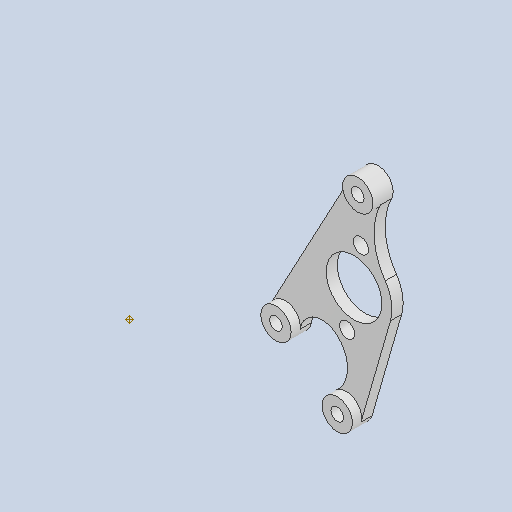
# Autodesk Inventor part: モータマウント
Saved by Autodesk Inventor 2023 (Build 270158030, 158C)
## iProperties
Created: 2022-01-29
Part Number: モータマウント
Material: Aluminum 2014-T4
Document SubType Name: Modeling
Designer: acps
Density: 2.8 g/cm^3
Appearance: Satin
Author: acps
Autodesk Inventor part; units mm, degrees
ref_plane "YZ Plane" through (0, 0, 0) normal (1, 0, 0) x (0, 1, 0)
ref_plane "XZ Plane" through (0, 0, 0) normal (0, 1, 0) x (-1, 0, 0)
ref_plane "XY Plane" through (0, 0, 0) normal (0, 0, 1) x (1, 0, 0)
sketch "Sketch1" plane through (0, 0, 0) normal (0, 0, 1) x (1, 0, 0)
  circle A0 centre (46.616, 30) radius 5.5
  circle A1 centre (49.1519, 48.073) radius 1.25
  circle A2 centre (45.1, 8.5) radius 1.25
  circle A3 centre (47.9747, 37.8838) radius 1.5
  line L0 (47.9747, 37.8838) -> (46.616, 30)
  line L1 (46.616, 30) -> (45.2573, 22.1162)
  circle A4 centre (45.2573, 22.1162) radius 2.75 construction
  circle A5 centre (33, 18) radius 1.25
  arc A6 (53.8224, 27.9221) -> (52.7865, 34.2633) centre (46.616, 30) ccw
  circle A7 centre (45.2573, 22.1162) radius 1.5
  circle A8 centre (49.1519, 48.073) radius 3
  circle A9 centre (33, 18) radius 3
  circle A10 centre (45.1, 8.5) radius 3
  arc A11 (51.8473, 46.7559) -> (52.7865, 34.2633) centre (62.9884, 41.3118) ccw
  arc A12 (43.1426, 10.7734) -> (43.3656, 20.1202) centre (39.0319, 15.5476) ccw
  arc A13 (43.3656, 20.1202) -> (35.9679, 17.5623) centre (40.3315, 16.9188) ccw
  line L2 (53.8224, 27.9221) -> (47.9826, 7.6688)
  line L3 (46.509, 49.4925) -> (30.3571, 19.4195)
  circle A14 centre (47.9747, 37.8838) radius 3 construction
  point P0 (0, 0)
  point P1 (0, 0)
  dimension "d65" = 5.5
  dimension "d61" = 11
  dimension "d62" = 3
  dimension "d63" = 8
  dimension "d64" = 8
  dimension "d66" = 2
  dimension "d67" = 3
  dimension "d68" = 6
  dimension "d69" = 6
  dimension "d70" = 6
  dimension "d71" = 6.3
  dimension "d72" = 12.4
  dimension "d73" = 1.5
  constraints: 14 centre point, 14 point on circle, 9 tangent, 8 end point, 6 coincident, 1 collinear, 1 concentric, 11 other
  measures "d61" diameter of A0
  measures "d62" diameter of A3
  measures "d63" distance of L0.start L0.end
  measures "d64" distance of L0.end L1.end
  measures "d66" radial gap between concentric circles of A6 A0
  measures "d67" diameter of A7
  measures "d68" diameter of A8
  measures "d69" diameter of A9
  measures "d70" diameter of A10
  measures "d71" radius of A12
  measures "d72" radius of A11
  measures "d73" radial gap between concentric circles of A3 A14
extrude "Extrusion5" add sketch "Sketch1" along normal blind 2.2 contours L2 A10 A12 A13 A9 L3 A8 A11 A6
extrude "Extrusion6" add sketch "Sketch1" along normal blind 4 contours A10 | A8 | A9
body "Solid2"
